Autodesk Inventor part; units mm, degrees
(part 2 of 2)
sketch "Sketch2" plane through (0, 0, 0) normal (0, 0, -1) x (-1, 0, 0)
  line L0 (36.3108, 151.145) -> (38.286, 150.8307) projected
  line L1 (38.286, 150.8307) -> (38.1088, 149.7177) projected
  arc A0 (36.1337, 150.032) -> (38.1088, 149.7177) centre (36.5125, 146.05) ccw projected
  line L2 (36.1337, 150.032) -> (36.3108, 151.145) projected
  arc A1 (35.8103, 125.4117) -> (36.3775, 122.9364) centre (44.6705, 126.1394) ccw projected
  arc A2 (36.3775, 122.9364) -> (37.6493, 122.964) centre (36.5125, 146.05) ccw projected
  arc A3 (37.6493, 122.964) -> (38.1087, 125.4616) centre (29.2253, 125.8045) ccw projected
  arc A4 (38.1087, 125.4616) -> (39.5067, 125.618) centre (36.5125, 146.05) ccw projected
  arc A5 (39.5067, 125.618) -> (40.5068, 123.2837) centre (48.0946, 127.916) ccw projected
  arc A6 (40.5068, 123.2837) -> (41.7532, 123.538) centre (36.5125, 146.05) ccw projected
  arc A7 (41.7532, 123.538) -> (41.7592, 126.0775) centre (32.9574, 124.8286) ccw projected
  arc A8 (41.7592, 126.0775) -> (43.1068, 126.481) centre (36.5125, 146.05) ccw projected
  arc A9 (43.1068, 126.481) -> (44.5077, 124.3628) centre (51.1464, 130.2755) ccw projected
  arc A10 (44.5077, 124.3628) -> (45.6887, 124.8355) centre (36.5125, 146.05) ccw projected
  arc A11 (45.6887, 124.8355) -> (45.2412, 127.3353) centre (36.8037, 124.5349) ccw projected
  arc A12 (45.2412, 127.3353) -> (46.4951, 127.973) centre (36.5125, 146.05) ccw projected
  arc A13 (46.4951, 127.973) -> (48.2516, 126.1389) centre (53.7278, 133.142) ccw projected
  arc A14 (48.2516, 126.1389) -> (49.3292, 126.8149) centre (36.5125, 146.05) ccw projected
  arc A15 (49.3292, 126.8149) -> (48.4425, 129.1946) centre (40.6407, 124.9326) ccw projected
  arc A16 (48.4425, 129.1946) -> (49.5624, 130.0459) centre (36.5125, 146.05) ccw projected
  arc A17 (49.5624, 130.0459) -> (51.6182, 128.555) centre (55.756, 136.4233) ccw projected
  arc A18 (51.6182, 128.555) -> (52.5578, 129.4125) centre (36.5125, 146.05) ccw projected
  arc A19 (52.5578, 129.4125) -> (51.2605, 131.5956) centre (44.345, 126.0091) ccw projected
  arc A20 (51.2605, 131.5956) -> (52.2103, 132.6333) centre (36.5125, 146.05) ccw projected
  arc A21 (52.2103, 132.6333) -> (54.4993, 131.5334) centre (57.1657, 140.0141) ccw projected
  arc A22 (54.4993, 131.5334) -> (55.2707, 132.5449) centre (36.5125, 146.05) ccw projected
  arc A23 (55.2707, 132.5449) -> (53.6044, 134.4613) centre (47.7976, 127.7298) ccw projected
  arc A24 (53.6044, 134.4613) -> (54.3537, 135.6518) centre (36.5125, 146.05) ccw projected
  arc A25 (54.3537, 135.6518) -> (56.8023, 134.9783) centre (57.9115, 143.7989) ccw projected
  arc A26 (56.8023, 134.9783) -> (57.3806, 136.1113) centre (36.5125, 146.05) ccw projected
  arc A27 (57.3806, 136.1113) -> (55.399, 137.6994) centre (50.8874, 130.0392) ccw projected
  arc A28 (55.399, 137.6994) -> (55.9237, 139.0046) centre (36.5125, 146.05) ccw projected
  arc A29 (55.9237, 139.0046) -> (58.4531, 138.7791) centre (57.9696, 147.656) ccw projected
  arc A30 (58.4531, 138.7791) -> (58.8199, 139.9972) centre (36.5125, 146.05) ccw projected
  arc A31 (58.8199, 139.9972) -> (56.5865, 141.2059) centre (53.5153, 132.8632) ccw projected
  arc A32 (56.5865, 141.2059) -> (56.8697, 142.5838) centre (36.5125, 146.05) ccw projected
  arc A33 (56.8697, 142.5838) -> (59.3988, 142.8136) centre (57.338, 151.4615) ccw projected
  arc A34 (59.3988, 142.8136) -> (59.5422, 144.0776) centre (36.5125, 146.05) ccw projected
  arc A35 (59.5422, 144.0776) -> (57.1288, 144.8681) centre (55.5966, 136.1111) ccw projected
  arc A36 (57.1288, 144.8681) -> (57.1615, 146.2744) centre (36.5125, 146.05) ccw projected
  arc A37 (57.1615, 146.2744) -> (59.6089, 146.9522) centre (56.037, 155.0931) ccw projected
  arc A38 (59.6089, 146.9522) -> (59.5243, 148.2214) centre (36.5125, 146.05) ccw projected
  arc A39 (59.5243, 148.2214) -> (57.0086, 148.5683) centre (57.0646, 139.6785) ccw projected
  arc A40 (57.0086, 148.5683) -> (56.7896, 149.9579) centre (36.5125, 146.05) ccw projected
  arc A41 (56.7896, 149.9579) -> (59.0766, 151.0617) centre (54.1086, 158.434) ccw projected
  arc A42 (59.0766, 151.0617) -> (58.7668, 152.2954) centre (36.5125, 146.05) ccw projected
  arc A43 (58.7668, 152.2954) -> (56.2295, 152.1875) centre (57.872, 143.4506) ccw projected
  arc A44 (56.2295, 152.1875) -> (55.7659, 153.5157) centre (36.5125, 146.05) ccw projected
  arc A45 (55.7659, 153.5157) -> (57.8191, 155.0101) centre (51.6146, 161.3769) ccw projected
  arc A46 (57.8191, 155.0101) -> (57.294, 156.1687) centre (36.5125, 146.05) ccw projected
  arc A47 (57.294, 156.1687) -> (54.8168, 155.6095) centre (57.9929, 147.3062) ccw projected
  arc A48 (54.8168, 155.6095) -> (54.1235, 156.8335) centre (36.5125, 146.05) ccw projected
  arc A49 (54.1235, 156.8335) -> (55.8768, 158.6706) centre (48.6352, 163.8271) ccw projected
  arc A50 (55.8768, 158.6706) -> (55.1532, 159.7168) centre (36.5125, 146.05) ccw projected
  arc A51 (55.1532, 159.7168) -> (52.8157, 158.7242) centre (57.4234, 151.1215) ccw projected
  arc A52 (52.8157, 158.7242) -> (51.915, 159.8048) centre (36.5125, 146.05) ccw projected
  arc A53 (51.915, 159.8048) -> (53.3122, 161.9254) centre (45.2661, 165.706) ccw projected
  arc A54 (53.3122, 161.9254) -> (52.4134, 162.8256) centre (36.5125, 146.05) ccw projected
  arc A55 (52.4134, 162.8256) -> (50.2906, 161.4316) centre (56.1818, 154.7738) ccw projected
  arc A56 (50.2906, 161.4316) -> (49.2114, 162.334) centre (36.5125, 146.05) ccw projected
  arc A57 (49.2114, 162.334) -> (50.2075, 164.67) centre (41.6157, 166.9532) ccw projected
  arc A58 (50.2075, 164.67) -> (49.1624, 165.3952) centre (36.5125, 146.05) ccw projected
  arc A59 (49.1624, 165.3952) -> (47.3227, 163.6446) centre (54.308, 158.1457) ccw projected
  arc A60 (47.3227, 163.6446) -> (46.0998, 164.3398) centre (36.5125, 146.05) ccw projected
  arc A61 (46.0998, 164.3398) -> (46.6627, 166.8161) centre (37.8013, 167.5284) ccw projected
  arc A62 (46.6627, 166.8161) -> (45.5049, 167.343) centre (36.5125, 146.05) ccw projected
  arc A63 (45.5049, 167.343) -> (44.0074, 165.2921) centre (51.8622, 161.1288) ccw projected
  arc A64 (44.0074, 165.2921) -> (42.6799, 165.7577) centre (36.5125, 146.05) ccw projected
  arc A65 (42.6799, 165.7577) -> (42.7917, 168.2948) centre (33.9455, 167.4134) ccw projected
  arc A66 (42.7917, 168.2948) -> (41.5584, 168.6065) centre (36.5125, 146.05) ccw projected
  arc A67 (41.5584, 168.6065) -> (40.4511, 166.3211) centre (48.9231, 163.6273) ccw projected
  arc A68 (40.4511, 166.3211) -> (39.0619, 166.5422) centre (36.5125, 146.05) ccw projected
  arc A69 (39.0619, 166.5422) -> (38.7188, 169.0585) centre (30.1721, 166.6117) ccw projected
  arc A70 (38.7188, 169.0585) -> (37.4497, 169.145) centre (36.5125, 146.05) ccw projected
  arc A71 (37.4497, 169.145) -> (36.7683, 166.6986) centre (45.5852, 165.5608) ccw projected
  arc A72 (36.7683, 166.6986) -> (35.3619, 166.6681) centre (36.5125, 146.05) ccw projected
  arc A73 (35.3619, 166.6681) -> (34.575, 169.0827) centre (26.6026, 165.1492) ccw projected
  arc A74 (34.575, 169.0827) -> (33.3109, 168.9412) centre (36.5125, 146.05) ccw projected
  arc A75 (33.3109, 168.9412) -> (33.0772, 166.4125) centre (41.9556, 166.8672) ccw projected
  arc A76 (33.0772, 166.4125) -> (31.6988, 166.1313) centre (36.5125, 146.05) ccw projected
  arc A77 (31.6988, 166.1313) -> (30.4935, 168.3666) centre (23.3516, 163.0728) ccw projected
  arc A78 (30.4935, 168.3666) -> (29.2749, 168.0016) centre (36.5125, 146.05) ccw projected
  arc A79 (29.2749, 168.0016) -> (29.4966, 165.4718) centre (38.151, 167.5046) ccw projected
  arc A80 (29.4966, 165.4718) -> (28.1905, 164.9491) centre (36.5125, 146.05) ccw projected
  arc A81 (28.1905, 164.9491) -> (26.6055, 166.9332) centre (20.5235, 160.4492) ccw projected
  arc A82 (26.6055, 166.9332) -> (25.4716, 166.3566) centre (36.5125, 146.05) ccw projected
  arc A83 (25.4716, 166.3566) -> (26.1414, 163.907) centre (34.2938, 167.4524) ccw projected
  arc A84 (26.1414, 163.907) -> (24.9497, 163.1594) centre (36.5125, 146.05) ccw projected
  arc A85 (24.9497, 163.1594) -> (23.0359, 164.8286) centre (18.2094, 157.3629) ccw projected
  arc A86 (23.0359, 164.8286) -> (22.0232, 164.0588) centre (36.5125, 146.05) ccw projected
  arc A87 (22.0232, 164.0588) -> (23.1196, 161.7682) centre (30.5079, 166.7123) ccw projected
  arc A88 (23.1196, 161.7682) -> (22.0805, 160.8199) centre (36.5125, 146.05) ccw projected
  arc A89 (22.0805, 160.8199) -> (19.8994, 162.1205) centre (16.4835, 153.9129) ccw projected
  arc A90 (19.8994, 162.1205) -> (19.0404, 161.1822) centre (36.5125, 146.05) ccw projected
  arc A91 (19.0404, 161.1822) -> (20.5282, 159.1242) centre (26.915, 165.3081) ccw projected
  arc A92 (20.5282, 159.1242) -> (19.6752, 158.0056) centre (36.5125, 146.05) ccw projected
  arc A93 (19.6752, 158.0056) -> (17.2969, 158.8959) centre (15.4014, 150.2103) ccw projected
  arc A94 (17.2969, 158.8959) -> (16.6193, 157.8193) centre (36.5125, 146.05) ccw projected
  arc A95 (16.6193, 157.8193) -> (18.4506, 156.06) centre (23.6306, 163.2849) ccw projected
  arc A96 (18.4506, 156.06) -> (17.811, 154.807) centre (36.5125, 146.05) ccw projected
  arc A97 (17.811, 154.807) -> (15.3119, 155.2583) centre (14.9979, 146.3739) ccw projected
  arc A98 (15.3119, 155.2583) -> (14.8375, 154.0781) centre (36.5125, 146.05) ccw projected
  arc A99 (14.8375, 154.0781) -> (16.9535, 152.674) centre (20.7602, 160.7078) ccw projected
  arc A100 (16.9535, 152.674) -> (16.5479, 151.327) centre (36.5125, 146.05) ccw projected
  arc A101 (16.5479, 151.327) -> (14.0084, 151.3248) centre (15.2858, 142.5271) ccw projected
  arc A102 (14.0084, 151.3248) -> (13.7523, 150.0788) centre (36.5125, 146.05) ccw projected
  arc A103 (13.7523, 150.0788) -> (16.0851, 149.0752) centre (18.3961, 157.6595) ccw projected
  arc A104 (16.0851, 149.0752) -> (15.9265, 147.6774) centre (36.5125, 146.05) ccw projected
  arc A105 (15.9265, 147.6774) -> (13.4282, 147.2218) centre (16.2559, 138.7935) ccw projected
  arc A106 (13.4282, 147.2218) -> (13.3987, 145.9501) centre (36.5125, 146.05) ccw projected
  arc A107 (13.3987, 145.9501) -> (15.8732, 145.3791) centre (16.6143, 154.2382) ccw projected
  arc A108 (15.8732, 145.3791) -> (15.9668, 143.9755) centre (36.5125, 146.05) ccw projected
  arc A109 (15.9668, 143.9755) -> (13.59, 143.0811) centre (17.8772, 135.2932) ccw projected
  arc A110 (13.59, 143.0811) -> (13.788, 141.8246) centre (36.5125, 146.05) ccw projected
  arc A111 (13.788, 141.8246) -> (16.3247, 141.7046) centre (15.472, 150.5536) ccw projected
  arc A112 (16.3247, 141.7046) -> (16.6674, 140.3403) centre (36.5125, 146.05) ccw projected
  arc A113 (16.6674, 140.3403) -> (14.4884, 139.0359) centre (20.0973, 132.1386) ccw projected
  arc A114 (14.4884, 139.0359) -> (14.9077, 137.8349) centre (36.5125, 146.05) ccw projected
  arc A115 (14.9077, 137.8349) -> (17.425, 138.1698) centre (15.006, 146.7243) ccw projected
  arc A116 (17.425, 138.1698) -> (18.0058, 136.8885) centre (36.5125, 146.05) ccw projected
  arc A117 (18.0058, 136.8885) -> (16.0948, 135.216) centre (22.8451, 129.4311) ccw projected
  arc A118 (16.0948, 135.216) -> (16.7217, 134.1092) centre (36.5125, 146.05) ccw projected
  arc A119 (16.7217, 134.1092) -> (19.1388, 134.8882) centre (15.2312, 142.8734) ccw projected
  arc A120 (19.1388, 134.8882) -> (19.9391, 133.7313) centre (36.5125, 146.05) ccw projected
  arc A121 (19.9391, 133.7313) -> (18.3574, 131.7444) centre (26.0322, 127.2578) ccw projected
  arc A122 (18.3574, 131.7444) -> (19.1719, 130.7673) centre (36.5125, 146.05) ccw projected
  arc A123 (19.1719, 130.7673) -> (21.411, 131.9654) centre (16.1404, 139.1245) ccw projected
  arc A124 (21.411, 131.9654) -> (22.405, 130.9699) centre (36.5125, 146.05) ccw projected
  arc A125 (22.405, 130.9699) -> (21.2035, 128.7326) centre (29.5561, 125.6884) ccw projected
  arc A126 (21.2035, 128.7326) -> (22.1794, 127.9166) centre (36.5125, 146.05) ccw projected
  arc A127 (22.1794, 127.9166) -> (24.1686, 129.4953) centre (17.7044, 135.5982) ccw projected
  arc A128 (24.1686, 129.4953) -> (25.3244, 128.6933) centre (36.5125, 146.05) ccw projected
  arc A129 (25.3244, 128.6933) -> (24.5417, 126.2774) centre (33.3036, 124.7735) ccw projected
  arc A130 (24.5417, 126.2774) -> (25.6476, 125.6488) centre (36.5125, 146.05) ccw projected
  arc A131 (25.6476, 125.6488) -> (27.323, 127.5572) centre (19.8729, 132.4078) ccw projected
  arc A132 (27.323, 127.5572) -> (28.6033, 126.9745) centre (36.5125, 146.05) ccw projected
  arc A133 (28.6033, 126.9745) -> (28.2646, 124.4577) centre (37.1542, 124.5425) ccw projected
  arc A134 (28.2646, 124.4577) -> (29.465, 124.0366) centre (36.5125, 146.05) ccw projected
  arc A135 (29.465, 124.0366) -> (30.7727, 126.2135) centre (22.5762, 129.656) ccw projected
  arc A136 (30.7727, 126.2135) -> (32.1365, 125.8688) centre (36.5125, 146.05) ccw projected
  arc A137 (32.1365, 125.8688) -> (32.2526, 123.3319) centre (40.9842, 125.0027) ccw projected
  arc A138 (32.2526, 123.3319) -> (33.5089, 123.132) centre (36.5125, 146.05) ccw projected
  arc A139 (33.5089, 123.132) -> (34.4068, 125.5074) centre (25.7274, 127.431) ccw projected
  arc A140 (34.4068, 125.5074) -> (35.8103, 125.4117) centre (36.5125, 146.05) ccw projected
  circle A141 centre (-6.6997, 178.392) radius 13.97 projected
  arc A142 (21.375, 167.3307) -> (24.3142, 167.0582) centre (24.0087, 179.7546) ccw projected
  arc A143 (24.3142, 167.0582) -> (24.6456, 168.0098) centre (-6.6997, 178.392) ccw projected
  arc A144 (24.6456, 168.0098) -> (22.1729, 169.6221) centre (16.5199, 158.2496) ccw projected
  arc A145 (22.1729, 169.6221) -> (22.5399, 170.9366) centre (-6.6997, 178.392) ccw projected
  arc A146 (22.5399, 170.9366) -> (25.4902, 171.0347) centre (23.5958, 183.5926) ccw projected
  arc A147 (25.4902, 171.0347) -> (25.6997, 172.0203) centre (-6.6997, 178.392) ccw projected
  arc A148 (25.6997, 172.0203) -> (23.0444, 173.3099) centre (18.8613, 161.3186) ccw projected
  arc A149 (23.0444, 173.3099) -> (23.2438, 174.6601) centre (-6.6997, 178.392) ccw projected
  arc A150 (23.2438, 174.6601) -> (26.1585, 175.1272) centre (22.7051, 187.3486) ccw projected
  arc A151 (26.1585, 175.1272) -> (26.2428, 176.1313) centre (-6.6997, 178.392) ccw projected
  arc A152 (26.2428, 176.1313) -> (23.4468, 177.0779) centre (20.7996, 164.6569) ccw projected
  arc A153 (23.4468, 177.0779) -> (23.4754, 178.4424) centre (-6.6997, 178.392) ccw projected
  arc A154 (23.4754, 178.4424) -> (26.3085, 179.2711) centre (21.3507, 190.9634) ccw projected
  arc A155 (26.3085, 179.2711) -> (26.2663, 180.2779) centre (-6.6997, 178.392) ccw projected
  arc A156 (26.2663, 180.2779) -> (23.3738, 180.8667) centre (22.3042, 168.2118) ccw projected
  arc A157 (23.3738, 180.8667) -> (23.2311, 182.224) centre (-6.6997, 178.392) ccw projected
  arc A158 (23.2311, 182.224) -> (25.9381, 183.4012) centre (19.5538, 194.3799) ccw projected
  arc A159 (25.9381, 183.4012) -> (25.77, 184.3948) centre (-6.6997, 178.392) ccw projected
  arc A160 (25.77, 184.3948) -> (22.8265, 184.6164) centre (23.3514, 171.9272) ccw projected
  arc A161 (22.8265, 184.6164) -> (22.5149, 185.9451) centre (-6.6997, 178.392) ccw projected
  arc A162 (22.5149, 185.9451) -> (25.0529, 187.4523) centre (17.343, 197.5443) ccw projected
  arc A163 (25.0529, 187.4523) -> (24.7616, 188.417) centre (-6.6997, 178.392) ccw projected
  arc A164 (24.7616, 188.417) -> (21.8136, 188.2679) centre (23.9247, 175.7446) ccw projected
  arc A165 (21.8136, 188.2679) -> (21.3378, 189.5471) centre (-6.6997, 178.392) ccw projected
  arc A166 (21.3378, 189.5471) -> (23.6669, 191.3606) centre (14.753, 200.4066) ccw projected
  arc A167 (23.6669, 191.3606) -> (23.2571, 192.2811) centre (-6.6997, 178.392) ccw projected
  arc A168 (23.2571, 192.2811) -> (20.3509, 191.7637) centre (24.015, 179.6037) ccw projected
  arc A169 (20.3509, 191.7637) -> (19.7186, 192.9732) centre (-6.6997, 178.392) ccw projected
  arc A170 (19.7186, 192.9732) -> (21.8021, 195.0643) centre (11.8247, 202.9218) ccw projected
  arc A171 (21.8021, 195.0643) -> (21.2801, 195.9262) centre (-6.6997, 178.392) ccw projected
  arc A172 (21.2801, 195.9262) -> (18.4617, 195.0486) centre (23.621, 183.4438) ccw projected
  arc A173 (18.4617, 195.0486) -> (17.6828, 196.1693) centre (-6.6997, 178.392) ccw projected
  arc A174 (17.6828, 196.1693) -> (19.4877, 198.505) centre (8.6042, 205.0501) ccw projected
  arc A175 (19.4877, 198.505) -> (18.8618, 199.2947) centre (-6.6997, 178.392) ccw projected
  arc A176 (18.8618, 199.2947) -> (16.1757, 198.0708) centre (22.7487, 187.2041) ccw projected
  arc A177 (16.1757, 198.0708) -> (15.2624, 199.0851) centre (-6.6997, 178.392) ccw projected
  arc A178 (15.2624, 199.0851) -> (16.7604, 201.6286) centre (5.1424, 206.758) ccw projected
  arc A179 (16.7604, 201.6286) -> (16.0405, 202.3336) centre (-6.6997, 178.392) ccw projected
  arc A180 (16.0405, 202.3336) -> (13.5289, 200.7827) centre (21.4121, 190.8255) ccw projected
  arc A181 (13.5289, 200.7827) -> (12.4957, 201.6745) centre (-6.6997, 178.392) ccw projected
  arc A182 (12.4957, 201.6745) -> (13.6631, 204.3857) centre (1.4938, 208.0185) ccw projected
  arc A183 (13.6631, 204.3857) -> (12.8605, 204.9949) centre (-6.6997, 178.392) ccw projected
  arc A184 (12.8605, 204.9949) -> (10.5631, 203.1415) centre (19.632, 194.2508) ccw projected
  arc A185 (10.5631, 203.1415) -> (9.4263, 203.8967) centre (-6.6997, 178.392) ccw projected
  arc A186 (9.4263, 203.8967) -> (10.2447, 206.7329) centre (-2.284, 208.8118) ccw projected
  arc A187 (10.2447, 206.7329) -> (9.372, 207.2367) centre (-6.6997, 178.392) ccw projected
  arc A188 (9.372, 207.2367) -> (7.325, 205.1099) centre (17.4368, 197.426) ccw projected
  arc A189 (7.325, 205.1099) -> (6.1025, 205.7167) centre (-6.6997, 178.392) ccw projected
  arc A190 (6.1025, 205.7167) -> (6.559, 208.6331) centre (-6.1315, 209.1254) ccw projected
  arc A191 (6.559, 208.6331) -> (5.6301, 209.0236) centre (-6.6997, 178.392) ccw projected
  arc A192 (5.6301, 209.0236) -> (3.8658, 206.657) centre (14.8608, 200.301) ccw projected
  arc A193 (3.8658, 206.657) -> (2.5769, 207.1058) centre (-6.6997, 178.392) ccw projected
  arc A194 (2.5769, 207.1058) -> (2.6642, 210.0564) centre (-9.9879, 208.9543) ccw projected
  arc A195 (2.6642, 210.0564) -> (1.6937, 210.3274) centre (-6.6997, 178.392) ccw projected
  arc A196 (1.6937, 210.3274) -> (0.2399, 207.7583) centre (11.9449, 202.8305) ccw projected
  arc A197 (0.2399, 207.7583) -> (-1.0951, 208.0421) centre (-6.6997, 178.392) ccw projected
  arc A198 (-1.0951, 208.0421) -> (-1.3782, 210.9803) centre (-13.7924, 208.3012) ccw projected
  arc A199 (-1.3782, 210.9803) -> (-2.3751, 211.1275) centre (-6.6997, 178.392) ccw projected
  arc A200 (-2.3751, 211.1275) -> (-3.4954, 208.3965) centre (8.7349, 204.9746) ccw projected
  arc A201 (-3.4954, 208.3965) -> (-4.8554, 208.5107) centre (-6.6997, 178.392) ccw projected
  arc A202 (-4.8554, 208.5107) -> (-5.5046, 211.3903) centre (-17.4851, 207.1764) ccw projected
  arc A203 (-5.5046, 211.3903) -> (-6.512, 211.4114) centre (-6.6997, 178.392) ccw projected
  arc A204 (-6.512, 211.4114) -> (-7.2812, 208.5616) centre (5.2815, 206.6995) ccw projected
  arc A205 (-7.2812, 208.5616) -> (-8.6448, 208.5044) centre (-6.6997, 178.392) ccw projected
  arc A206 (-8.6448, 208.5044) -> (-9.6498, 211.2799) centre (-21.0077, 205.5976) ccw projected
  arc A207 (-9.6498, 211.2799) -> (-10.6519, 211.1746) centre (-6.6997, 178.392) ccw projected
  arc A208 (-10.6519, 211.1746) -> (-11.0579, 208.2508) centre (1.6392, 207.9779) ccw projected
  arc A209 (-11.0579, 208.2508) -> (-12.4036, 208.0232) centre (-6.6997, 178.392) ccw projected
  arc A210 (-12.4036, 208.0232) -> (-13.7485, 210.6508) centre (-24.3047, 203.5899) ccw projected
  arc A211 (-13.7485, 210.6508) -> (-14.7295, 210.4207) centre (-6.6997, 178.392) ccw projected
  arc A212 (-14.7295, 210.4207) -> (-14.7658, 207.4691) centre (-2.1347, 208.7898) ccw projected
  arc A213 (-14.7658, 207.4691) -> (-16.0724, 207.0746) centre (-6.6997, 178.392) ccw projected
  arc A214 (-16.0724, 207.0746) -> (-17.736, 209.513) centre (-27.324, 201.1847) ccw projected
  arc A215 (-17.736, 209.513) -> (-18.6805, 209.1618) centre (-6.6997, 178.392) ccw projected
  arc A216 (-18.6805, 209.1618) -> (-18.3466, 206.2289) centre (-5.9806, 209.1222) ccw projected
  arc A217 (-18.3466, 206.2289) -> (-19.5934, 205.6738) centre (-6.6997, 178.392) ccw projected
  arc A218 (-19.5934, 205.6738) -> (-21.5495, 207.8844) centre (-30.018, 198.4201) ccw projected
  arc A219 (-21.5495, 207.8844) -> (-22.4425, 207.4176) centre (-6.6997, 178.392) ccw projected
  arc A220 (-22.4425, 207.4176) -> (-21.7436, 204.5496) centre (-9.8377, 208.9701) ccw projected
  arc A221 (-21.7436, 204.5496) -> (-22.911, 203.8426) centre (-6.6997, 178.392) ccw projected
  arc A222 (-22.911, 203.8426) -> (-25.1288, 205.7907) centre (-32.3443, 195.3396) ccw projected
  arc A223 (-25.1288, 205.7907) -> (-25.9562, 205.2156) centre (-6.6997, 178.392) ccw projected
  arc A224 (-25.9562, 205.2156) -> (-24.9034, 202.4579) centre (-13.6455, 208.3356) ccw projected
  arc A225 (-24.9034, 202.4579) -> (-25.973, 201.6101) centre (-6.6997, 178.392) ccw projected
  arc A226 (-25.973, 201.6101) -> (-28.4175, 203.2649) centre (-34.2662, 191.9918) ccw projected
  arc A227 (-28.4175, 203.2649) -> (-29.1663, 202.5906) centre (-6.6997, 178.392) ccw projected
  arc A228 (-29.1663, 202.5906) -> (-27.7761, 199.9866) centre (-17.3436, 207.229) ccw projected
  arc A229 (-27.7761, 199.9866) -> (-28.731, 199.0115) centre (-6.6997, 178.392) ccw projected
  arc A230 (-28.731, 199.0115) -> (-31.3636, 200.3468) centre (-35.7534, 188.4296) ccw projected
  arc A231 (-31.3636, 200.3468) -> (-32.022, 199.584) centre (-6.6997, 178.392) ccw projected
  arc A232 (-32.022, 199.584) -> (-30.3165, 197.1747) centre (-20.8739, 205.6676) ccw projected
  arc A233 (-30.3165, 197.1747) -> (-31.1416, 196.0876) centre (-6.6997, 178.392) ccw projected
  arc A234 (-31.1416, 196.0876) -> (-33.9208, 197.0825) centre (-36.7823, 184.709) ccw projected
  arc A235 (-33.9208, 197.0825) -> (-34.4784, 196.2432) centre (-6.6997, 178.392) ccw projected
  arc A236 (-34.4784, 196.2432) -> (-32.4844, 194.0667) centre (-24.1807, 203.676) ccw projected
  arc A237 (-32.4844, 194.0667) -> (-33.1668, 192.8847) centre (-6.6997, 178.392) ccw projected
  arc A238 (-33.1668, 192.8847) -> (-36.0487, 193.5234) centre (-37.3369, 180.8889) ccw projected
  arc A239 (-36.0487, 193.5234) -> (-36.4967, 192.6208) centre (-6.6997, 178.392) ccw projected
  arc A240 (-36.4967, 192.6208) -> (-34.2456, 190.7114) centre (-27.2118, 201.2857) ccw projected
  arc A241 (-34.2456, 190.7114) -> (-34.7745, 189.4533) centre (-6.6997, 178.392) ccw projected
  arc A242 (-34.7745, 189.4533) -> (-37.7137, 189.7257) centre (-37.4082, 177.0293) ccw projected
  arc A243 (-37.7137, 189.7257) -> (-38.0451, 188.7741) centre (-6.6997, 178.392) ccw projected
  arc A244 (-38.0451, 188.7741) -> (-35.5724, 187.1618) centre (-29.9194, 198.5343) ccw projected
  arc A245 (-35.5724, 187.1618) -> (-35.9394, 185.8473) centre (-6.6997, 178.392) ccw projected
  arc A246 (-35.9394, 185.8473) -> (-38.8897, 185.7492) centre (-36.9953, 173.1913) ccw projected
  arc A247 (-38.8897, 185.7492) -> (-39.0992, 184.7636) centre (-6.6997, 178.392) ccw projected
  arc A248 (-39.0992, 184.7636) -> (-36.4439, 183.474) centre (-32.2608, 195.4653) ccw projected
  arc A249 (-36.4439, 183.474) -> (-36.6433, 182.1238) centre (-6.6997, 178.392) ccw projected
  arc A250 (-36.6433, 182.1238) -> (-39.558, 181.6567) centre (-36.1046, 169.4353) ccw projected
  arc A251 (-39.558, 181.6567) -> (-39.6423, 180.6526) centre (-6.6997, 178.392) ccw projected
  arc A252 (-39.6423, 180.6526) -> (-36.8463, 179.706) centre (-34.1991, 192.127) ccw projected
  arc A253 (-36.8463, 179.706) -> (-36.8749, 178.3415) centre (-6.6997, 178.392) ccw projected
  arc A254 (-36.8749, 178.3415) -> (-39.708, 177.5128) centre (-34.7502, 165.8205) ccw projected
  arc A255 (-39.708, 177.5128) -> (-39.6658, 176.506) centre (-6.6997, 178.392) ccw projected
  arc A256 (-39.6658, 176.506) -> (-36.7733, 175.9172) centre (-35.7037, 188.5721) ccw projected
  arc A257 (-36.7733, 175.9172) -> (-36.6306, 174.5599) centre (-6.6997, 178.392) ccw projected
  arc A258 (-36.6306, 174.5599) -> (-39.3376, 173.3827) centre (-32.9533, 162.404) ccw projected
  arc A259 (-39.3376, 173.3827) -> (-39.1695, 172.3891) centre (-6.6997, 178.392) ccw projected
  arc A260 (-39.1695, 172.3891) -> (-36.226, 172.1675) centre (-36.7509, 184.8567) ccw projected
  arc A261 (-36.226, 172.1675) -> (-35.9143, 170.8388) centre (-6.6997, 178.392) ccw projected
  arc A262 (-35.9143, 170.8388) -> (-38.4524, 169.3316) centre (-30.7425, 159.2396) ccw projected
  arc A263 (-38.4524, 169.3316) -> (-38.1611, 168.3669) centre (-6.6997, 178.392) ccw projected
  arc A264 (-38.1611, 168.3669) -> (-35.2131, 168.516) centre (-37.3242, 181.0393) ccw projected
  arc A265 (-35.2131, 168.516) -> (-34.7373, 167.2368) centre (-6.6997, 178.392) ccw projected
  arc A266 (-34.7373, 167.2368) -> (-37.0664, 165.4233) centre (-28.1525, 156.3773) ccw projected
  arc A267 (-37.0664, 165.4233) -> (-36.6566, 164.5028) centre (-6.6997, 178.392) ccw projected
  arc A268 (-36.6566, 164.5028) -> (-33.7504, 165.0202) centre (-37.4145, 177.1802) ccw projected
  arc A269 (-33.7504, 165.0202) -> (-33.1181, 163.8107) centre (-6.6997, 178.392) ccw projected
  arc A270 (-33.1181, 163.8107) -> (-35.2016, 161.7197) centre (-25.2242, 153.8621) ccw projected
  arc A271 (-35.2016, 161.7197) -> (-34.6796, 160.8577) centre (-6.6997, 178.392) ccw projected
  arc A272 (-34.6796, 160.8577) -> (-31.8612, 161.7353) centre (-37.0205, 173.3401) ccw projected
  arc A273 (-31.8612, 161.7353) -> (-31.0823, 160.6146) centre (-6.6997, 178.392) ccw projected
  arc A274 (-31.0823, 160.6146) -> (-32.8872, 158.2789) centre (-22.0037, 151.7338) ccw projected
  arc A275 (-32.8872, 158.2789) -> (-32.2613, 157.4892) centre (-6.6997, 178.392) ccw projected
  arc A276 (-32.2613, 157.4892) -> (-29.5752, 158.7131) centre (-36.1482, 169.5798) ccw projected
  arc A277 (-29.5752, 158.7131) -> (-28.6619, 157.6989) centre (-6.6997, 178.392) ccw projected
  arc A278 (-28.6619, 157.6989) -> (-30.1599, 155.1553) centre (-18.5419, 150.0259) ccw projected
  arc A279 (-30.1599, 155.1553) -> (-29.44, 154.4503) centre (-6.6997, 178.392) ccw projected
  arc A280 (-29.44, 154.4503) -> (-26.9284, 156.0012) centre (-34.8116, 165.9584) ccw projected
  arc A281 (-26.9284, 156.0012) -> (-25.8952, 155.1094) centre (-6.6997, 178.392) ccw projected
  arc A282 (-25.8952, 155.1094) -> (-27.0626, 152.3982) centre (-14.8933, 148.7654) ccw projected
  arc A283 (-27.0626, 152.3982) -> (-26.26, 151.789) centre (-6.6997, 178.392) ccw projected
  arc A284 (-26.26, 151.789) -> (-23.9626, 153.6424) centre (-33.0315, 162.5331) ccw projected
  arc A285 (-23.9626, 153.6424) -> (-22.8258, 152.8872) centre (-6.6997, 178.392) ccw projected
  arc A286 (-22.8258, 152.8872) -> (-23.6442, 150.051) centre (-11.1155, 147.9721) ccw projected
  arc A287 (-23.6442, 150.051) -> (-22.7715, 149.5472) centre (-6.6997, 178.392) ccw projected
  arc A288 (-22.7715, 149.5472) -> (-20.7245, 151.674) centre (-30.8363, 159.3579) ccw projected
  arc A289 (-20.7245, 151.674) -> (-19.502, 151.0672) centre (-6.6997, 178.392) ccw projected
  arc A290 (-19.502, 151.0672) -> (-19.9585, 148.1508) centre (-7.268, 147.6585) ccw projected
  arc A291 (-19.9585, 148.1508) -> (-19.0296, 147.7603) centre (-6.6997, 178.392) ccw projected
  arc A292 (-19.0296, 147.7603) -> (-17.2653, 150.1269) centre (-28.2603, 156.4829) ccw projected
  arc A293 (-17.2653, 150.1269) -> (-15.9764, 149.6781) centre (-6.6997, 178.392) ccw projected
  arc A294 (-15.9764, 149.6781) -> (-16.0637, 146.7275) centre (-3.4116, 147.8296) ccw projected
  arc A295 (-16.0637, 146.7275) -> (-15.0932, 146.4565) centre (-6.6997, 178.392) ccw projected
  arc A296 (-15.0932, 146.4565) -> (-13.6394, 149.0256) centre (-25.3444, 153.9534) ccw projected
  arc A297 (-13.6394, 149.0256) -> (-12.3044, 148.7418) centre (-6.6997, 178.392) ccw projected
  arc A298 (-12.3044, 148.7418) -> (-12.0213, 145.8036) centre (0.3929, 148.4827) ccw projected
  arc A299 (-12.0213, 145.8036) -> (-11.0244, 145.6564) centre (-6.6997, 178.392) ccw projected
  arc A300 (-11.0244, 145.6564) -> (-9.9041, 148.3874) centre (-22.1344, 151.8093) ccw projected
  arc A301 (-9.9041, 148.3874) -> (-8.5441, 148.2732) centre (-6.6997, 178.392) ccw projected
  arc A302 (-8.5441, 148.2732) -> (-7.8949, 145.3936) centre (4.0856, 149.6075) ccw projected
  arc A303 (-7.8949, 145.3936) -> (-6.8875, 145.3725) centre (-6.6997, 178.392) ccw projected
  arc A304 (-6.8875, 145.3725) -> (-6.1183, 148.2224) centre (-18.681, 150.0844) ccw projected
  arc A305 (-6.1183, 148.2224) -> (-4.7547, 148.2795) centre (-6.6997, 178.392) ccw projected
  arc A306 (-4.7547, 148.2795) -> (-3.7497, 145.504) centre (7.6082, 151.1863) ccw projected
  arc A307 (-3.7497, 145.504) -> (-2.7476, 145.6093) centre (-6.6997, 178.392) ccw projected
  arc A308 (-2.7476, 145.6093) -> (-2.3416, 148.5331) centre (-15.0387, 148.806) ccw projected
  arc A309 (-2.3416, 148.5331) -> (-0.9959, 148.7607) centre (-6.6997, 178.392) ccw projected
  arc A310 (-0.9959, 148.7607) -> (0.349, 146.1331) centre (10.9052, 153.1941) ccw projected
  arc A311 (0.349, 146.1331) -> (1.33, 146.3632) centre (-6.6997, 178.392) ccw projected
  arc A312 (1.33, 146.3632) -> (1.3663, 149.3148) centre (-11.2648, 147.9941) ccw projected
  arc A313 (1.3663, 149.3148) -> (2.6729, 149.7093) centre (-6.6997, 178.392) ccw projected
  arc A314 (2.6729, 149.7093) -> (4.3365, 147.2709) centre (13.9245, 155.5992) ccw projected
  arc A315 (4.3365, 147.2709) -> (5.281, 147.6221) centre (-6.6997, 178.392) ccw projected
  arc A316 (5.281, 147.6221) -> (4.9471, 150.555) centre (-7.4189, 147.6617) ccw projected
  arc A317 (4.9471, 150.555) -> (6.1939, 151.1101) centre (-6.6997, 178.392) ccw projected
  arc A318 (6.1939, 151.1101) -> (8.15, 148.8995) centre (16.6185, 158.3639) ccw projected
  arc A319 (8.15, 148.8995) -> (9.043, 149.3663) centre (-6.6997, 178.392) ccw projected
  arc A320 (9.043, 149.3663) -> (8.3441, 152.2343) centre (-3.5618, 147.8139) ccw projected
  arc A321 (8.3441, 152.2343) -> (9.5115, 152.9413) centre (-6.6997, 178.392) ccw projected
  arc A322 (9.5115, 152.9413) -> (11.7293, 150.9932) centre (18.9448, 161.4443) ccw projected
  arc A323 (11.7293, 150.9932) -> (12.5567, 151.5683) centre (-6.6997, 178.392) ccw projected
  arc A324 (12.5567, 151.5683) -> (11.5039, 154.326) centre (0.246, 148.4483) ccw projected
  arc A325 (11.5039, 154.326) -> (12.5735, 155.1738) centre (-6.6997, 178.392) ccw projected
  arc A326 (12.5735, 155.1738) -> (15.018, 153.519) centre (20.8667, 164.7921) ccw projected
  arc A327 (15.018, 153.519) -> (15.7668, 154.1933) centre (-6.6997, 178.392) ccw projected
  arc A328 (15.7668, 154.1933) -> (14.3766, 156.7973) centre (3.9441, 149.5549) ccw projected
  arc A329 (14.3766, 156.7973) -> (15.3315, 157.7724) centre (-6.6997, 178.392) ccw projected
  arc A330 (15.3315, 157.7724) -> (17.9641, 156.4371) centre (22.3539, 168.3543) ccw projected
  arc A331 (17.9641, 156.4371) -> (18.6225, 157.1999) centre (-6.6997, 178.392) ccw projected
  arc A332 (18.6225, 157.1999) -> (16.917, 159.6092) centre (7.4744, 151.1163) ccw projected
  arc A333 (16.917, 159.6092) -> (17.7421, 160.6963) centre (-6.6997, 178.392) ccw projected
  arc A334 (17.7421, 160.6963) -> (20.5213, 159.7014) centre (23.3828, 172.0749) ccw projected
  arc A335 (20.5213, 159.7014) -> (21.0789, 160.5407) centre (-6.6997, 178.392) ccw projected
  arc A336 (21.0789, 160.5407) -> (19.0849, 162.7172) centre (10.7812, 153.1079) ccw projected
  arc A337 (19.0849, 162.7172) -> (19.7673, 163.8992) centre (-6.6997, 178.392) ccw projected
  arc A338 (19.7673, 163.8992) -> (22.6492, 163.2605) centre (23.9374, 175.895) ccw projected
  arc A339 (22.6492, 163.2605) -> (23.0972, 164.1631) centre (-6.6997, 178.392) ccw projected
  arc A340 (23.0972, 164.1631) -> (20.8461, 166.0725) centre (13.8123, 155.4982) ccw projected
  arc A341 (20.8461, 166.0725) -> (21.375, 167.3307) centre (-6.6997, 178.392) ccw projected
  line L3 (61.9125, 171.704) -> (29.446, 168.6111) projected
  circle A342 centre (-6.6997, 178.392) radius 37.4457
  circle A343 centre (36.5125, 146.05) radius 28.194
  point P0 (0, 0)
  point P1 (50.3685, 170.6043)
  point P2 (30.4357, 173.5813)
  dimension "d10" = 56.388
  constraints: 2 coincident, 1 centre point, 3 other
  measures "d10" diameter of A343
extrude "Extrusion2" cut sketch "Sketch2" against normal blind 12.7 contours A343 L3 A342
sketch "Sketch3" plane through (0, 0, 0) normal (0, 0, -1) x (-1, 0, 0)
  arc A0 (50.3685, 170.6043) -> (30.6784, 173.6338) centre (36.5125, 146.05) ccw projected
  line L0 (61.9125, 171.704) -> (50.3685, 170.6043) projected
  line L1 (61.9125, 190.5) -> (61.9125, 171.704) projected
  arc A1 (37.5415, 269.5562) -> (-0.498, 236.0395) centre (17.4625, 254) ccw projected
  circle A2 centre (17.4625, 254) radius 15.9004 projected
  circle A3 centre (40.0964, 179.0237) radius 3.175 projected
  circle A4 centre (52.7964, 180.2336) radius 3.175 projected
  circle A5 centre (40.0964, 182.1987) radius 3.175
  point P0 (0, 0)
  point P1 (42.8461, 180.6112)
  point P2 (37.3468, 180.6112)
  dimension "d13" = 6.35
  constraints: 1 centre point, 4 other
  measures "d13" diameter of A5
extrude "Extrusion3" add sketch "Sketch3" against normal blind 12.7 contours A3 A5 picked at (39.9369, 176.9303)
extrude "Extrusion4" cut sketch "Sketch3" against normal blind 12.7 contours A3 A5 picked at (39.9369, 184.2921)
fillet "Fillet1" radius 6.35 3 edges at (-30.6784, 173.6338, 6.35) (-50.3685, 170.6043, 6.35) (-61.9125, 171.704, 6.35)
sketch "Sketch4" plane through (0, 0, 0) normal (0, 0, -1) x (-1, 0, 0)
  arc A0 (56.1647, 171.1564) -> (61.9125, 177.4778) centre (55.5625, 177.4778) ccw projected
  line L0 (61.9125, 190.5) -> (61.9125, 177.4778) projected
  spline S0 degree 2 poles (37.5415, 269.5562) (61.9125, 238.0996) (61.9125, 190.5) knots 0 0 0 1 1 1
  arc A1 (37.5415, 269.5562) -> (-0.498, 236.0395) centre (17.4625, 254) ccw projected
  spline S1 degree 3 poles (31.1263, 180.4076) (30.6021, 199.6374) (15.5371, 220.0043) (-0.498, 236.0395) knots 0 0 0 0 1 1 1 1
  arc A2 (48.8612, 171.3959) -> (37.2972, 174.2331) centre (36.5125, 146.05) ccw projected
  arc A3 (48.8612, 171.3959) -> (52.2446, 170.783) centre (51.6424, 177.1044) ccw projected
  line L1 (56.1647, 171.1564) -> (52.2446, 170.783) projected
  circle A4 centre (17.4625, 254) radius 15.9004 projected
  circle A5 centre (40.0964, 182.1987) radius 3.175 projected
  circle A6 centre (52.7964, 180.2336) radius 3.175 projected
  line L2 (55.5625, 190.5) -> (55.5625, 177.4778)
  line L3 (55.5625, 177.4778) -> (51.6424, 177.1044)
  arc A7 (51.6424, 177.1044) -> (37.4739, 180.5806) centre (36.5125, 146.05) ccw
  arc A8 (32.5217, 265.6671) -> (3.9921, 240.5296) centre (17.4625, 254) ccw
  circle A9 centre (17.4625, 254) radius 25.4
  circle A10 centre (40.0964, 182.1987) radius 9.525
  circle A11 centre (52.7964, 180.2336) radius 9.525
  line L4 (35.7519, 192.1076) -> (55.5625, 190.5)
  line L5 (42.5378, 249.9517) -> (35.7519, 192.1076)
  line L6 (46.3219, 249.5078) -> (39.9961, 195.5857)
  line L7 (39.9961, 195.5857) -> (59.3725, 194.0133)
  line L8 (59.3725, 194.0133) -> (59.3725, 174.0135)
  line L9 (59.3725, 174.0135) -> (50.9032, 173.2067)
  arc A12 (50.9032, 173.2067) -> (37.3679, 176.7721) centre (36.5125, 146.05) ccw
  line L10 (40.0134, 250.2478) -> (32.9205, 189.7873)
  line L11 (32.9205, 189.7873) -> (53.0208, 188.1562)
  line L12 (53.0208, 188.1562) -> (53.0208, 179.7889)
  line L13 (53.0208, 179.7889) -> (52.0994, 179.7012)
  arc A13 (52.0994, 179.7012) -> (37.5447, 183.1214) centre (36.5125, 146.05) ccw
  spline S2 degree 5 poles (37.4739, 180.5806) (37.3509, 185.1082) (36.6509, 189.6212) (35.4639, 194.0199) (32.2784, 202.7446) (27.8412, 210.9069) (25.3327, 214.9313) (19.904, 222.7569) (13.835, 230.0962) (10.658, 233.6733) (7.3727, 237.149) (3.9921, 240.5296) knots 0 0 0 0 0 0 0.3225 0.3225 0.3225 0.6596 0.6596 0.6596 1 1 1 1 1 1
  spline S3 degree 5 poles (32.5217, 265.6671) (37.1582, 259.6822) (41.243, 253.2684) (44.699, 246.4805) (50.6714, 231.5564) (53.993, 215.8141) (55.0644, 207.401) (55.5628, 198.9509) (55.5625, 190.5) knots 0 0 0 0 0 0 0.472546 0.472546 0.472546 1 1 1 1 1 1
  point P0 (0, 0)
  point P1 (33.8801, 197.967)
  point P2 (38.8453, 240.2911)
  point P3 (14.8615, 228.7335)
  point P4 (55.5211, 194.3259)
  point P5 (45.6111, 243.4492)
  dimension "d19" = 6.35
  dimension "d20" = 19.05
  dimension "d21" = 19.05
  dimension "d22" = 3.81
  constraints: 24 end point, 8 point on circle, 6 centre point, 3 coincident, 3 concentric, 1 tangent, 24 other
  measures "d20" diameter of A10
  measures "d21" diameter of A11
  measures "d22" distance between parallel lines of L5 L6
extrude "Extrusion5" cut sketch "Sketch4" against normal blind 12.7 contours L7 L6 S3 | A9 L10 S2
fillet "Fillet2" radius 3.175 6 edges at (-38.8453, 240.2911, 6.35) (-45.6111, 243.4492, 6.35) (-14.8615, 228.7335, 6.35) (-33.8801, 197.967, 6.35) (-39.9961, 195.5857, 6.35) (-55.5212, 194.3259, 6.35)
thread "Thread1" size "1/4-20 UNC" class "2B" standard "ANSI Unified Screw Threads" full length
thread "Thread2" size "8-32 UNC" class "2B" standard "ANSI Unified Screw Threads" full length
sketch "Sketch5" plane through (0, 0, 0) normal (0, 0, -1) x (-1, 0, 0)
  circle A0 centre (52.7964, 180.2336) radius 3.175 projected
  circle A1 centre (52.7964, 180.2336) radius 2.413
  circle A2 centre (40.0964, 182.1987) radius 3.175 projected
  circle A3 centre (40.0964, 182.1987) radius 2.413
  point P0 (0, 0)
  dimension "d30" = 4.826
  dimension "d31" = 4.826
  constraints: 2 centre point, 2 coincident
  measures "d30" diameter of A1
  measures "d31" diameter of A3
extrude "Extrusion6" add sketch "Sketch5" against normal blind 12.7
thread "Thread3" size "10-24 UNC" class "2B" standard "ANSI Unified Screw Threads" full length
thread "Thread4" size "10-24 UNC" class "2B" standard "ANSI Unified Screw Threads" full length
sketch "Sketch6" plane through (0, 0, 12.7) normal (0, 0, 1) x (1, 0, 0)
  circle A0 centre (-40.0964, 182.1987) radius 2.413 projected
  circle A1 centre (-52.7964, 180.2336) radius 2.413 projected
  line L0 (-35.1978, 209.1987) -> (-37.7252, 230.7434) projected
  arc A2 (-32.6708, 233.6563) -> (-37.7252, 230.7434) centre (-34.5719, 231.1133) ccw projected
  arc A3 (-32.6708, 233.6563) -> (-20.9604, 228.842) centre (-17.4625, 254) ccw projected
  line L1 (-44.0388, 230.0468) -> (-40.3795, 198.8541) projected
  arc A4 (-43.2761, 195.3195) -> (-40.3795, 198.8541) centre (-43.5329, 198.4841) ccw projected
  line L2 (-43.2761, 195.3195) -> (-51.9761, 194.6136) projected
  arc A5 (-61.9125, 177.4778) -> (-56.1647, 171.1564) centre (-55.5625, 177.4778) ccw projected
  line L3 (-56.1647, 171.1564) -> (-52.2446, 170.783) projected
  arc A6 (-52.2446, 170.783) -> (-48.8612, 171.3959) centre (-51.6424, 177.1044) ccw projected
  arc A7 (-37.2972, 174.2331) -> (-48.8612, 171.3959) centre (-36.5125, 146.05) ccw projected
  arc A8 (0.498, 236.0395) -> (-37.5415, 269.5562) centre (-17.4625, 254) ccw projected
  line L4 (-61.9125, 190.5) -> (-61.9125, 177.4778) projected
  circle A9 centre (-17.4625, 254) radius 15.9004 projected
  circle A10 centre (-52.7964, 180.2336) radius 1.27
  circle A11 centre (-40.0964, 182.1987) radius 1.27
  point P0 (0, 0)
  dimension "d38" = 2.54
  dimension "d39" = 2.54
  constraints: 2 centre point, 2 coincident, 9 other
  measures "d38" diameter of A10
  measures "d39" diameter of A11
extrude "Extrusion7" add sketch "Sketch6" against normal up to surface (12.7 mm away) contours A0 | A1
sketch "Sketch7" plane through (0, 0, 12.7) normal (0, 0, 1) x (1, 0, 0)
  circle A0 centre (-40.0964, 182.1987) radius 1.27 projected
  circle A1 centre (-52.7964, 180.2336) radius 1.27 projected
  line L0 (-35.1978, 209.1987) -> (-37.7252, 230.7434) projected
  arc A2 (-32.6708, 233.6563) -> (-37.7252, 230.7434) centre (-34.5719, 231.1133) ccw projected
  arc A3 (-32.6708, 233.6563) -> (-20.9604, 228.842) centre (-17.4625, 254) ccw projected
  line L1 (-44.0388, 230.0468) -> (-40.3795, 198.8541) projected
  arc A4 (-43.2761, 195.3195) -> (-40.3795, 198.8541) centre (-43.5329, 198.4841) ccw projected
  line L2 (-43.2761, 195.3195) -> (-51.9761, 194.6136) projected
  arc A5 (-61.9125, 177.4778) -> (-56.1647, 171.1564) centre (-55.5625, 177.4778) ccw projected
  line L3 (-56.1647, 171.1564) -> (-52.2446, 170.783) projected
  arc A6 (-52.2446, 170.783) -> (-48.8612, 171.3959) centre (-51.6424, 177.1044) ccw projected
  arc A7 (-37.2972, 174.2331) -> (-48.8612, 171.3959) centre (-36.5125, 146.05) ccw projected
  arc A8 (0.498, 236.0395) -> (-37.5415, 269.5562) centre (-17.4625, 254) ccw projected
  line L4 (-61.9125, 190.5) -> (-61.9125, 177.4778) projected
  circle A9 centre (-17.4625, 254) radius 15.9004 projected
  circle A10 centre (-17.4625, 254) radius 15.24
  point P0 (0, 0)
  dimension "d42" = 30.48
  constraints: 1 centre point, 1 coincident, 9 other
  measures "d42" diameter of A10
extrude "Extrusion8" add sketch "Sketch7" against normal blind 12.7 contours A9
body "Solid1"
